Autodesk Inventor part; units mm, degrees
(part 2 of 2)
  line L503 (-41.6487, 6.565) -> (-41.6409, 7.3338) construction
  line L504 (-41.6409, 7.3338) -> (-41.6386, 7.5646) construction
  line L505 (-41.6386, 7.5646) -> (-41.6931, 7.6742) construction
  line L506 (-41.6931, 7.6742) -> (-41.9588, 7.6723) construction
  line L507 (-41.9588, 7.6723) -> (-42.2269, 7.6704) construction
  line L508 (-42.2269, 7.6704) -> (-42.3043, 7.5774) construction
  line L509 (-42.3043, 7.5774) -> (-42.3018, 7.3204) construction
  line L510 (-42.3018, 7.3204) -> (-42.2917, 6.2568) construction
  line L511 (-42.2917, 6.2568) -> (-42.2958, 5.193) construction
  line L512 (-42.2958, 5.193) -> (-42.2984, 4.1292) construction
  line L513 (-42.2984, 4.1292) -> (-42.3, 3.4632) construction
  line L514 (-42.3, 3.4632) -> (-42.5495, 3.2131) construction
  line L515 (-42.5495, 3.2131) -> (-43.2106, 3.2105) construction
  line L516 (-43.2106, 3.2105) -> (-43.8425, 3.2081) construction
  line L517 (-43.8425, 3.2081) -> (-44.4746, 3.2036) construction
  line L518 (-44.4746, 3.2036) -> (-45.1064, 3.2123) construction
  line L519 (-45.1064, 3.2123) -> (-45.7637, 3.2212) construction
  line L520 (-45.7637, 3.2212) -> (-46.0284, 3.4861) construction
  line L521 (-46.0284, 3.4861) -> (-46.0307, 4.1394) construction
  line L522 (-46.0307, 4.1394) -> (-46.0356, 5.498) construction
  line L523 (-46.0356, 5.498) -> (-46.0352, 6.8567) construction
  line L524 (-46.0352, 6.8567) -> (-46.0307, 8.2153) construction
  line L525 (-46.0307, 8.2153) -> (-46.0284, 8.8905) construction
  line L526 (-46.0284, 8.8905) -> (-45.7896, 9.1207) construction
  line L527 (-45.7896, 9.1207) -> (-45.1112, 9.1248) construction
  line L528 (-45.1112, 9.1248) -> (-44.8291, 9.1265) construction
  line L529 (-44.8291, 9.1265) -> (-44.547, 9.1251) construction
  line L530 (-44.547, 9.1251) -> (-44.2474, 9.1251) construction
  spline S8 degree 3 poles (-43.0206, -3.033) (-43.6937, -3.0331) (-44.3669, -3.0367) (-45.04, -3.0321) (-45.6795, -3.0278) (-46.0304, -2.6732) (-46.0317, -2.0319) (-46.0341, -0.8118) (-46.0336, 0.4082) (-46.0319, 1.6283) (-46.031, 2.2514) (-45.631, 2.6629) (-45.0162, 2.6647) (-43.6909, 2.6685) (-42.3657, 2.6688) (-41.0405, 2.6645) (-40.3992, 2.6624) (-40.0861, 2.3514) (-40.0845, 1.7196) (-40.0811, 0.447) (-40.0811, -0.8257) (-40.0845, -2.0983) (-40.0862, -2.7432) (-40.3593, -3.0232) (-41.0012, -3.031) (-41.6742, -3.0392) (-42.3474, -3.0328) (-43.0206, -3.033) knots 0 0 0 0 1 1 1 2 2 2 3 3 3 4 4 4 5 5 5 6 6 6 7 7 7 8 8 8 9 9 9 9
  line L531 (-43.0206, -3.033) -> (-43.6937, -3.0331) construction
  line L532 (-43.6937, -3.0331) -> (-44.3669, -3.0367) construction
  line L533 (-44.3669, -3.0367) -> (-45.04, -3.0321) construction
  line L534 (-45.04, -3.0321) -> (-45.6795, -3.0278) construction
  line L535 (-45.6795, -3.0278) -> (-46.0304, -2.6732) construction
  line L536 (-46.0304, -2.6732) -> (-46.0317, -2.0319) construction
  line L537 (-46.0317, -2.0319) -> (-46.0341, -0.8118) construction
  line L538 (-46.0341, -0.8118) -> (-46.0336, 0.4082) construction
  line L539 (-46.0336, 0.4082) -> (-46.0319, 1.6283) construction
  line L540 (-46.0319, 1.6283) -> (-46.031, 2.2514) construction
  line L541 (-46.031, 2.2514) -> (-45.631, 2.6629) construction
  line L542 (-45.631, 2.6629) -> (-45.0162, 2.6647) construction
  line L543 (-45.0162, 2.6647) -> (-43.6909, 2.6685) construction
  line L544 (-43.6909, 2.6685) -> (-42.3657, 2.6688) construction
  line L545 (-42.3657, 2.6688) -> (-41.0405, 2.6645) construction
  line L546 (-41.0405, 2.6645) -> (-40.3992, 2.6624) construction
  line L547 (-40.3992, 2.6624) -> (-40.0861, 2.3514) construction
  line L548 (-40.0861, 2.3514) -> (-40.0845, 1.7196) construction
  line L549 (-40.0845, 1.7196) -> (-40.0811, 0.447) construction
  line L550 (-40.0811, 0.447) -> (-40.0811, -0.8257) construction
  line L551 (-40.0811, -0.8257) -> (-40.0845, -2.0983) construction
  line L552 (-40.0845, -2.0983) -> (-40.0862, -2.7432) construction
  line L553 (-40.0862, -2.7432) -> (-40.3593, -3.0232) construction
  line L554 (-40.3593, -3.0232) -> (-41.0012, -3.031) construction
  line L555 (-41.0012, -3.031) -> (-41.6742, -3.0392) construction
  line L556 (-41.6742, -3.0392) -> (-42.3474, -3.0328) construction
  line L557 (-42.3474, -3.0328) -> (-43.0206, -3.033) construction
  spline S9 degree 3 poles (-41.6026, -1.5634) (-41.6026, -0.6351) (-41.6026, 0.2538) (-41.6026, 1.167) (-42.5619, 1.167) (-43.5004, 1.167) (-44.4345, 1.167) (-44.4345, 0.2444) (-44.4345, -0.6556) (-44.4345, -1.5634) (-43.4844, -1.5634) (-42.5538, -1.5634) (-41.6026, -1.5634) knots 0 0 0 0 1 1 1 2 2 2 3 3 3 4 4 4 4
  line L558 (-41.6026, -1.5634) -> (-41.6026, -0.6351) construction
  line L559 (-41.6026, -0.6351) -> (-41.6026, 0.2538) construction
  line L560 (-41.6026, 0.2538) -> (-41.6026, 1.167) construction
  line L561 (-41.6026, 1.167) -> (-42.5619, 1.167) construction
  line L562 (-42.5619, 1.167) -> (-43.5004, 1.167) construction
  line L563 (-43.5004, 1.167) -> (-44.4345, 1.167) construction
  line L564 (-44.4345, 1.167) -> (-44.4345, 0.2444) construction
  line L565 (-44.4345, 0.2444) -> (-44.4345, -0.6556) construction
  line L566 (-44.4345, -0.6556) -> (-44.4345, -1.5634) construction
  line L567 (-44.4345, -1.5634) -> (-43.4844, -1.5634) construction
  line L568 (-43.4844, -1.5634) -> (-42.5538, -1.5634) construction
  line L569 (-42.5538, -1.5634) -> (-41.6026, -1.5634) construction
  spline S10 degree 3 poles (-46.0019, -16.1978) (-46.0019, -15.7578) (-46.0019, -15.3412) (-46.0019, -14.8935) (-45.8811, -14.8876) (-45.7697, -14.8778) (-45.6582, -14.8776) (-44.7741, -14.8763) (-43.8893, -14.8563) (-43.006, -14.882) (-41.8875, -14.9147) (-41.3239, -14.0121) (-41.3775, -13.241) (-41.4438, -12.2885) (-42.3658, -11.593) (-43.3179, -11.7553) (-43.9795, -11.8681) (-44.7205, -12.3188) (-44.6453, -13.3103) (-44.6169, -13.6853) (-44.6407, -14.0643) (-44.6407, -14.4608) (-45.1001, -14.4608) (-45.5366, -14.4608) (-45.9953, -14.4608) (-45.9953, -13.1051) (-45.9953, -11.7534) (-45.9953, -10.378) (-44.032, -10.378) (-42.0717, -10.378) (-40.0922, -10.378) (-40.0922, -12.3189) (-40.0922, -14.2497) (-40.0922, -16.1978) (-42.0581, -16.1978) (-44.0121, -16.1978) (-46.0019, -16.1978) knots 0 0 0 0 1 1 1 2 2 2 3 3 3 4 4 4 5 5 5 6 6 6 7 7 7 8 8 8 9 9 9 10 10 10 11 11 11 12 12 12 12
  line L570 (-46.0019, -16.1978) -> (-46.0019, -15.7578) construction
  line L571 (-46.0019, -15.7578) -> (-46.0019, -15.3412) construction
  line L572 (-46.0019, -15.3412) -> (-46.0019, -14.8935) construction
  line L573 (-46.0019, -14.8935) -> (-45.8811, -14.8876) construction
  line L574 (-45.8811, -14.8876) -> (-45.7697, -14.8778) construction
  line L575 (-45.7697, -14.8778) -> (-45.6582, -14.8776) construction
  line L576 (-45.6582, -14.8776) -> (-44.7741, -14.8763) construction
  line L577 (-44.7741, -14.8763) -> (-43.8893, -14.8563) construction
  line L578 (-43.8893, -14.8563) -> (-43.006, -14.882) construction
  line L579 (-43.006, -14.882) -> (-41.8875, -14.9147) construction
  line L580 (-41.8875, -14.9147) -> (-41.3239, -14.0121) construction
  line L581 (-41.3239, -14.0121) -> (-41.3775, -13.241) construction
  line L582 (-41.3775, -13.241) -> (-41.4438, -12.2885) construction
  line L583 (-41.4438, -12.2885) -> (-42.3658, -11.593) construction
  line L584 (-42.3658, -11.593) -> (-43.3179, -11.7553) construction
  line L585 (-43.3179, -11.7553) -> (-43.9795, -11.8681) construction
  line L586 (-43.9795, -11.8681) -> (-44.7205, -12.3188) construction
  line L587 (-44.7205, -12.3188) -> (-44.6453, -13.3103) construction
  line L588 (-44.6453, -13.3103) -> (-44.6169, -13.6853) construction
  line L589 (-44.6169, -13.6853) -> (-44.6407, -14.0643) construction
  line L590 (-44.6407, -14.0643) -> (-44.6407, -14.4608) construction
  line L591 (-44.6407, -14.4608) -> (-45.1001, -14.4608) construction
  line L592 (-45.1001, -14.4608) -> (-45.5366, -14.4608) construction
  line L593 (-45.5366, -14.4608) -> (-45.9953, -14.4608) construction
  line L594 (-45.9953, -14.4608) -> (-45.9953, -13.1051) construction
  line L595 (-45.9953, -13.1051) -> (-45.9953, -11.7534) construction
  line L596 (-45.9953, -11.7534) -> (-45.9953, -10.378) construction
  line L597 (-45.9953, -10.378) -> (-44.032, -10.378) construction
  line L598 (-44.032, -10.378) -> (-42.0717, -10.378) construction
  line L599 (-42.0717, -10.378) -> (-40.0922, -10.378) construction
  line L600 (-40.0922, -10.378) -> (-40.0922, -12.3189) construction
  line L601 (-40.0922, -12.3189) -> (-40.0922, -14.2497) construction
  line L602 (-40.0922, -14.2497) -> (-40.0922, -16.1978) construction
  line L603 (-40.0922, -16.1978) -> (-42.0581, -16.1978) construction
  line L604 (-42.0581, -16.1978) -> (-44.0121, -16.1978) construction
  line L605 (-44.0121, -16.1978) -> (-46.0019, -16.1978) construction
  spline S11 degree 3 poles (-45.1707, -13.9968) (-45.1707, -13.7305) (-45.1718, -13.49) (-45.1705, -13.2494) (-45.165, -12.1812) (-44.4343, -11.3766) (-43.3407, -11.2337) (-42.2226, -11.0875) (-41.3199, -11.6499) (-41.0153, -12.6716) (-40.6188, -14.0019) (-41.5606, -15.4445) (-42.9983, -15.3476) (-43.3966, -15.3208) (-43.7982, -15.3436) (-44.1983, -15.3436) (-44.6266, -15.3436) (-45.0549, -15.3436) (-45.4875, -15.3436) (-45.4875, -15.4894) (-45.4875, -15.5964) (-45.4875, -15.6995) (-43.8239, -15.6995) (-42.1858, -15.6995) (-40.5438, -15.6995) (-40.5438, -14.077) (-40.5438, -12.4737) (-40.5438, -10.866) (-42.2046, -10.866) (-43.8421, -10.866) (-45.4914, -10.866) (-45.4914, -11.9179) (-45.4914, -12.9527) (-45.4914, -13.9968) (-45.3865, -13.9968) (-45.3042, -13.9968) (-45.1707, -13.9968) knots 0 0 0 0 1 1 1 2 2 2 3 3 3 4 4 4 5 5 5 6 6 6 7 7 7 8 8 8 9 9 9 10 10 10 11 11 11 12 12 12 12
  line L606 (-45.1707, -13.9968) -> (-45.1707, -13.7305) construction
  line L607 (-45.1707, -13.7305) -> (-45.1718, -13.49) construction
  line L608 (-45.1718, -13.49) -> (-45.1705, -13.2494) construction
  line L609 (-45.1705, -13.2494) -> (-45.165, -12.1812) construction
  line L610 (-45.165, -12.1812) -> (-44.4343, -11.3766) construction
  line L611 (-44.4343, -11.3766) -> (-43.3407, -11.2337) construction
  line L612 (-43.3407, -11.2337) -> (-42.2226, -11.0875) construction
  line L613 (-42.2226, -11.0875) -> (-41.3199, -11.6499) construction
  line L614 (-41.3199, -11.6499) -> (-41.0153, -12.6716) construction
  line L615 (-41.0153, -12.6716) -> (-40.6188, -14.0019) construction
  line L616 (-40.6188, -14.0019) -> (-41.5606, -15.4445) construction
  line L617 (-41.5606, -15.4445) -> (-42.9983, -15.3476) construction
  line L618 (-42.9983, -15.3476) -> (-43.3966, -15.3208) construction
  line L619 (-43.3966, -15.3208) -> (-43.7982, -15.3436) construction
  line L620 (-43.7982, -15.3436) -> (-44.1983, -15.3436) construction
  line L621 (-44.1983, -15.3436) -> (-44.6266, -15.3436) construction
  line L622 (-44.6266, -15.3436) -> (-45.0549, -15.3436) construction
  line L623 (-45.0549, -15.3436) -> (-45.4875, -15.3436) construction
  line L624 (-45.4875, -15.3436) -> (-45.4875, -15.4894) construction
  line L625 (-45.4875, -15.4894) -> (-45.4875, -15.5964) construction
  line L626 (-45.4875, -15.5964) -> (-45.4875, -15.6995) construction
  line L627 (-45.4875, -15.6995) -> (-43.8239, -15.6995) construction
  line L628 (-43.8239, -15.6995) -> (-42.1858, -15.6995) construction
  line L629 (-42.1858, -15.6995) -> (-40.5438, -15.6995) construction
  line L630 (-40.5438, -15.6995) -> (-40.5438, -14.077) construction
  line L631 (-40.5438, -14.077) -> (-40.5438, -12.4737) construction
  line L632 (-40.5438, -12.4737) -> (-40.5438, -10.866) construction
  line L633 (-40.5438, -10.866) -> (-42.2046, -10.866) construction
  line L634 (-42.2046, -10.866) -> (-43.8421, -10.866) construction
  line L635 (-43.8421, -10.866) -> (-45.4914, -10.866) construction
  line L636 (-45.4914, -10.866) -> (-45.4914, -11.9179) construction
  line L637 (-45.4914, -11.9179) -> (-45.4914, -12.9527) construction
  line L638 (-45.4914, -12.9527) -> (-45.4914, -13.9968) construction
  line L639 (-45.4914, -13.9968) -> (-45.3865, -13.9968) construction
  line L640 (-45.3865, -13.9968) -> (-45.3042, -13.9968) construction
  line L641 (-45.3042, -13.9968) -> (-45.1707, -13.9968) construction
  spline S12 degree 3 poles (-41.6026, -1.5634) (-42.5538, -1.5634) (-43.4844, -1.5634) (-44.4345, -1.5634) (-44.4345, -0.6556) (-44.4345, 0.2444) (-44.4345, 1.167) (-43.5004, 1.167) (-42.5619, 1.167) (-41.6026, 1.167) (-41.6026, 0.2538) (-41.6026, -0.6351) (-41.6026, -1.5634) knots 0 0 0 0 1 1 1 2 2 2 3 3 3 4 4 4 4
  line L642 (-41.6026, -1.5634) -> (-42.5538, -1.5634) construction
  line L643 (-42.5538, -1.5634) -> (-43.4844, -1.5634) construction
  line L644 (-43.4844, -1.5634) -> (-44.4345, -1.5634) construction
  line L645 (-44.4345, -1.5634) -> (-44.4345, -0.6556) construction
  line L646 (-44.4345, -0.6556) -> (-44.4345, 0.2444) construction
  line L647 (-44.4345, 0.2444) -> (-44.4345, 1.167) construction
  line L648 (-44.4345, 1.167) -> (-43.5004, 1.167) construction
  line L649 (-43.5004, 1.167) -> (-42.5619, 1.167) construction
  line L650 (-42.5619, 1.167) -> (-41.6026, 1.167) construction
  line L651 (-41.6026, 1.167) -> (-41.6026, 0.2538) construction
  line L652 (-41.6026, 0.2538) -> (-41.6026, -0.6351) construction
  line L653 (-41.6026, -0.6351) -> (-41.6026, -1.5634) construction
  spline S13 degree 3 poles (-45.1707, -13.9968) (-45.3042, -13.9968) (-45.3865, -13.9968) (-45.4914, -13.9968) (-45.4914, -12.9527) (-45.4914, -11.9179) (-45.4914, -10.866) (-43.8421, -10.866) (-42.2046, -10.866) (-40.5438, -10.866) (-40.5438, -12.4737) (-40.5438, -14.077) (-40.5438, -15.6995) (-42.1858, -15.6995) (-43.8239, -15.6995) (-45.4875, -15.6995) (-45.4875, -15.5964) (-45.4875, -15.4894) (-45.4875, -15.3436) (-45.0549, -15.3436) (-44.6266, -15.3436) (-44.1983, -15.3436) (-43.7982, -15.3436) (-43.3966, -15.3208) (-42.9983, -15.3476) (-41.5606, -15.4445) (-40.6188, -14.0019) (-41.0153, -12.6716) (-41.3199, -11.6499) (-42.2226, -11.0875) (-43.3407, -11.2337) (-44.4343, -11.3766) (-45.165, -12.1812) (-45.1705, -13.2494) (-45.1718, -13.49) (-45.1707, -13.7305) (-45.1707, -13.9968) knots 0 0 0 0 1 1 1 2 2 2 3 3 3 4 4 4 5 5 5 6 6 6 7 7 7 8 8 8 9 9 9 10 10 10 11 11 11 12 12 12 12
  line L654 (-45.1707, -13.9968) -> (-45.3042, -13.9968) construction
  line L655 (-45.3042, -13.9968) -> (-45.3865, -13.9968) construction
  line L656 (-45.3865, -13.9968) -> (-45.4914, -13.9968) construction
  line L657 (-45.4914, -13.9968) -> (-45.4914, -12.9527) construction
  line L658 (-45.4914, -12.9527) -> (-45.4914, -11.9179) construction
  line L659 (-45.4914, -11.9179) -> (-45.4914, -10.866) construction
  line L660 (-45.4914, -10.866) -> (-43.8421, -10.866) construction
  line L661 (-43.8421, -10.866) -> (-42.2046, -10.866) construction
  line L662 (-42.2046, -10.866) -> (-40.5438, -10.866) construction
  line L663 (-40.5438, -10.866) -> (-40.5438, -12.4737) construction
  line L664 (-40.5438, -12.4737) -> (-40.5438, -14.077) construction
  line L665 (-40.5438, -14.077) -> (-40.5438, -15.6995) construction
  line L666 (-40.5438, -15.6995) -> (-42.1858, -15.6995) construction
  line L667 (-42.1858, -15.6995) -> (-43.8239, -15.6995) construction
  line L668 (-43.8239, -15.6995) -> (-45.4875, -15.6995) construction
  line L669 (-45.4875, -15.6995) -> (-45.4875, -15.5964) construction
  line L670 (-45.4875, -15.5964) -> (-45.4875, -15.4894) construction
  line L671 (-45.4875, -15.4894) -> (-45.4875, -15.3436) construction
  line L672 (-45.4875, -15.3436) -> (-45.0549, -15.3436) construction
  line L673 (-45.0549, -15.3436) -> (-44.6266, -15.3436) construction
  line L674 (-44.6266, -15.3436) -> (-44.1983, -15.3436) construction
  line L675 (-44.1983, -15.3436) -> (-43.7982, -15.3436) construction
  line L676 (-43.7982, -15.3436) -> (-43.3966, -15.3208) construction
  line L677 (-43.3966, -15.3208) -> (-42.9983, -15.3476) construction
  line L678 (-42.9983, -15.3476) -> (-41.5606, -15.4445) construction
  line L679 (-41.5606, -15.4445) -> (-40.6188, -14.0019) construction
  line L680 (-40.6188, -14.0019) -> (-41.0153, -12.6716) construction
  line L681 (-41.0153, -12.6716) -> (-41.3199, -11.6499) construction
  line L682 (-41.3199, -11.6499) -> (-42.2226, -11.0875) construction
  line L683 (-42.2226, -11.0875) -> (-43.3407, -11.2337) construction
  line L684 (-43.3407, -11.2337) -> (-44.4343, -11.3766) construction
  line L685 (-44.4343, -11.3766) -> (-45.165, -12.1812) construction
  line L686 (-45.165, -12.1812) -> (-45.1705, -13.2494) construction
  line L687 (-45.1705, -13.2494) -> (-45.1718, -13.49) construction
  line L688 (-45.1718, -13.49) -> (-45.1707, -13.7305) construction
  line L689 (-45.1707, -13.7305) -> (-45.1707, -13.9968) construction
  point P0 (0, 0)
  constraints: 22 other
extrude "Extrusion4" add sketch "Sketch4" along normal blind 0.508
equation "\"d2\" = 0.5 * d1"
equation "\"d3\" = 0.5 * d0"
equation "\"d15\" = 0.5 * d12"
equation "\"d21\" = 0.5 * d20"
equation "\"d1\" = 60.325"
equation "\"d0\" = 114.3"
body "Solid1"
